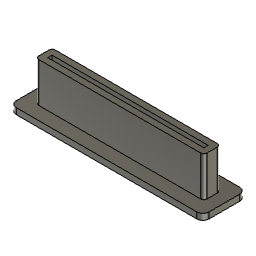
Grating_Holder v2 (Autodesk Fusion 360 design; units mm, degrees)
Autodesk Fusion 360 part; units mm, degrees
sketch "Sketch1" plane through (0, 0, 0) normal (0, 0, 1) x (1, 0, 0)
  line L0 (31.5, -7) -> (-31.5, -7)
  line L1 (-31.5, -7) -> (-31.5, 7)
  line L2 (-31.5, 7) -> (31.5, 7)
  line L3 (31.5, 7) -> (31.5, -7)
  line L4 (31.5, -7) -> (-31.5, 7) construction
  line L5 (-31.5, -7) -> (31.5, 7) construction
  dimension "d1" = 63
  dimension "d2" = 14
  constraint horizontal L0
  constraint perpendicular L0 L1
  constraint parallel L0 L2
  constraint parallel L1 L3
  constraint coincident L4 origin
  constraint coincident L5 origin
  measures "d1" distance of L1.end L2.end
  measures "d2" distance of L0.end L1.end
extrude "Extrude1" add sketch "Sketch1" along normal blind 2 makes body 1
sketch "Sketch3" plane through (0, 0, 2) normal (0, 0, 1) x (-1, 0, 0)
  line L0 (-31.5, -7) -> (31.5, -7)
  line L1 (31.5, -7) -> (31.5, 7)
  line L2 (31.5, 7) -> (-31.5, 7)
  line L3 (-31.5, 7) -> (-31.5, -7)
  line L4 (25.5, 0.7) -> (-25.5, 0.7)
  line L5 (-25.5, 0.7) -> (-25.5, -0.7)
  line L6 (-25.5, -0.7) -> (25.5, -0.7)
  line L7 (25.5, -0.7) -> (25.5, 0.7)
  line L8 (25.5, 0.7) -> (-25.5, -0.7) construction
  line L9 (-25.5, 0.7) -> (25.5, -0.7) construction
  line L10 (-27.5, 2.7) -> (27.5, 2.7)
  line L11 (27.5, 2.7) -> (27.5, -2.7)
  line L12 (27.5, -2.7) -> (-27.5, -2.7)
  line L13 (-27.5, -2.7) -> (-27.5, 2.7)
  line L14 (-27.5, 2.7) -> (27.5, -2.7) construction
  line L15 (27.5, 2.7) -> (-27.5, -2.7) construction
  dimension "d7" = 51
  dimension "d8" = 1.4
  dimension "d9" = 55
  dimension "d10" = 5.4
  constraint horizontal L4
  constraint perpendicular L4 L5
  constraint parallel L4 L6
  constraint parallel L5 L7
  constraint coincident L8 origin
  constraint coincident L9 origin
  constraint horizontal L10
  constraint perpendicular L10 L11
  constraint parallel L10 L12
  constraint parallel L11 L13
  constraint coincident L14 origin
  constraint coincident L15 origin
  measures "d7" distance of L5.end L6.end
  measures "d8" distance of L4.end L5.end
  measures "d9" distance of L11.end L12.end
  measures "d10" distance of L10.end L11.end
extrude "Extrude2" add sketch "Sketch3" along normal blind 13 contours L10 L11 L12 L13 bodies 1
fillet "Fillet1" radius 1 4 edges at (-27.5, -2.7, 8.5) (27.5, -2.7, 8.5) (-27.5, 2.7, 8.5) (27.5, 2.7, 8.5) on bodies 1
fillet "Fillet2" radius 2 4 edges at (-31.5, 7, 1) (31.5, 7, 1) (31.5, -7, 1) (-31.5, -7, 1) on bodies 1
copy_body "Body->Comp1" bodies 1 removing the originals makes body 2 in component "Grating_Holder"
component "Grating_Holder" placed x (1, 0, 0) y (0, 1, 0) z (0, 0, 1) at (0, 0, 0)
